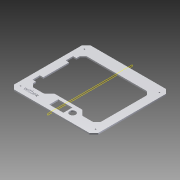
# Autodesk Inventor part: D-047
Saved by Autodesk Inventor 2015 (Build 190159000, 159)
## iProperties
Company: MARCHA TECHNOLOGY
Created: 2013-10-01
Part Number: D-047
Document SubType Name: Modeling
Designer: O.Martin
Density: 1.06 g/cm^3
Material: ABS Plastic
Mass: 736.814 g
Surface Area: 2028.63 cm^2
Volume: 695.108 cm^3
Project: WITBOXprinter_K01
Description: FRONTAL
Stock Number: 28655
Appearance: Cool White
Author: O.Martin
Autodesk Inventor part; units mm, degrees
ref_plane "XZ Plane" through (0, 0, 0) normal (0, 1, 0) x (-1, 0, 0)
ref_plane "XY Plane" through (0, 0, 0) normal (0, 0, 1) x (1, 0, 0)
sketch "Boceto1" plane through (0, 0, 0) normal (0, 0, 1) x (1, 0, 0)
  line L0 (-240, 218.25) -> (240, 218.25)
  line L1 (240, 218.25) -> (240, -218.25)
  line L2 (240, -218.25) -> (-240, -218.25)
  line L3 (-240, -218.25) -> (-240, 218.25)
  line L4 (-172.5, 153.25) -> (172.5, 153.25)
  line L5 (172.5, -153.25) -> (-172.5, -153.25)
  line L6 (-192.5, -133.25) -> (-192.5, 133.25)
  line L7 (172.5, 153.25) -> (192.5, 133.25)
  line L8 (-192.5, -133.25) -> (-172.5, -153.25)
  line L9 (-192.5, 133.25) -> (-172.5, 153.25)
  line L10 (-240, 193.25) -> (-215, 218.25)
  line L11 (240, 193.25) -> (215, 218.25)
  line L12 (-240, -193.25) -> (-215, -218.25)
  line L13 (240, -193.25) -> (215, -218.25)
  line L14 (192.5, -133.25) -> (192.5, 133.25)
  line L15 (-110, -153.25) -> (-80, -123.25)
  line L16 (-80, -123.25) -> (80, -123.25)
  line L17 (80, -123.25) -> (110, -153.25)
  line L18 (172.5, -153.25) -> (192.5, -133.25)
  point P0 (0, 0)
  point P1 (0, 218.25)
  point P2 (240, 0)
  point P3 (0, 153.25)
  point P4 (0, -123.25)
  point P5 (0, -153.25)
  point P6 (0, -218.25)
  dimension "d0" = 480
  dimension "d1" = 436.5
  dimension "d2" = 385
  dimension "d4" = 65
  dimension "d8" = 20
  dimension "d9" = 25
  dimension "d52" = 65
  dimension "d55" = 306.5
  dimension "d81" = 45
  dimension "d82" = 95
  dimension "d83" = 160
  dimension "d86" = 45
  constraints: 38 end point, 10 point on line, 7 parallel, 6 midpoint, 6 perpendicular, 5 equal length, 4 vertical alignment, 3 horizontal, 1 horizontal alignment, 1 vertical
  measures "d0" distance of L0.start L0.end
  measures "d1" distance of L0.end L1.end
  measures "d2" distance of L6.end L7.end
  measures "d4" distance between parallel lines of L2 L5
  measures "d8" horizontal distance of L6.end L4.start
  measures "d9" horizontal distance of L10.start L10.end
  measures "d52" distance between parallel lines of L0 L4
  measures "d55" distance between parallel lines of L4 L5
  measures "d81" angle of L2 L8
  measures "d82" distance between parallel lines of L2 L16
  measures "d83" distance of L15.end L16.end
  measures "d86" angle of L5 L15
extrude "Extrusión1" add sketch "Boceto1" along normal blind 8 contours L0 L11 L1 L13 L2 L12 L3 L10 | L15 L16 L17 L5
fillet "Empalme1" radius 10 12 edges at (192.5, 133.25, 4) (172.5, 153.25, 4) (-172.5, 153.25, 4) (-192.5, 133.25, 4) (-192.5, -133.25, 4) (-172.5, -153.25, 4) (-110, -153.25, 4) (110, -153.25, 4) (172.5, -153.25, 4) (192.5, -133.25, 4) (-80, -123.25, 4) (80, -123.25, 4)
sketch "Boceto3" plane through (0, 0, 8) normal (0, 0, 1) x (1, 0, 0)
  line L0 (-40.5, -141.25) -> (40.5, -141.25)
  line L1 (40.5, -141.25) -> (40.5, -192.25)
  line L2 (40.5, -192.25) -> (-40.5, -192.25)
  line L3 (-40.5, -192.25) -> (-40.5, -141.25)
  line L4 (215, -218.25) -> (-215, -218.25) projected
  line L5 (-40.5, -166.75) -> (40.5, -166.75) construction
  line L6 (0, -141.25) -> (0, -192.25) construction
  point P0 (0, -218.25)
  point P1 (0, -218.25)
  dimension "d32" = 81
  dimension "d33" = 51
  dimension "d102" = 51.5
  constraints: 12 end point, 5 midpoint, 2 parallel, 2 perpendicular, 2 vertical alignment, 1 horizontal
  measures "d32" distance of L1.end L2.end
  measures "d33" distance of L0.end L1.end
  measures "d102" distance between parallel lines of L4 L5
extrude "Extrusión3" cut sketch "Boceto3" against normal through all
sketch "Boceto8" plane through (0, 0, 8) normal (0, 0, 1) x (1, 0, 0)
  line L0 (40.5, -141.25) -> (40.5, -192.25) projected
  circle A0 centre (67.5, -166.75) radius 17.5
  line L1 (-40.5, -192.25) -> (-40.5, -141.25) projected
  line L2 (40.5, -166.75) -> (-40.5, -166.75) construction
  line L3 (-40.5, -141.25) -> (40.5, -141.25) projected
  line L4 (40.5, -192.25) -> (-40.5, -192.25) projected
  line L5 (0, -141.25) -> (0, -192.25) construction
  point P0 (190, -135.75)
  point P1 (171.2, -154.55)
  point P2 (190, -141.4069)
  dimension "d45" = 35
  dimension "d103" = 0
  dimension "d104" = 67.5
  constraints: 4 end point, 3 midpoint, 1 centre point, 2 other
  measures "d45" diameter of A0
  measures "d103" distance from line of A0.centre L2
  measures "d104" distance from line of A0.centre L5
extrude "Extrusión6" cut sketch "Boceto8" against normal through all contours A0
fillet "Empalme2" radius 1 4 edges at (-40.5, -192.25, 4) (40.5, -192.25, 4) (40.5, -141.25, 4) (-40.5, -141.25, 4)
sketch "Boceto10" plane through (0, 0, 0) normal (0, 0, -1) x (-1, 0, 0)
  line L0 (192.5, 129.1079) -> (192.5, -129.1079) projected
  line L1 (215, -218.25) -> (-215, -218.25) projected
  line L2 (192.5, 114.75) -> (211.5, 114.75)
  line L3 (211.5, 114.75) -> (211.5, 72.75)
  line L4 (211.5, 72.75) -> (192.5, 72.75)
  line L5 (192.5, 72.75) -> (192.5, 114.75)
  line L6 (192.5, -74.75) -> (211.5, -74.75)
  line L7 (211.5, -74.75) -> (211.5, -116.75)
  line L8 (211.5, -116.75) -> (192.5, -116.75)
  line L9 (192.5, -116.75) -> (192.5, -74.75)
  line L10 (211.5, -95.75) -> (192.5, -95.75) construction
  line L11 (211.5, 93.75) -> (192.5, 93.75) construction
  dimension "d60" = 42
  dimension "d61" = 122.5
  dimension "d62" = 19
  dimension "d63" = 189.5
  constraints: 20 end point, 4 midpoint, 4 parallel, 2 equal length, 2 horizontal, 2 perpendicular, 2 point on line
  measures "d60" distance of L6.end L7.end
  measures "d61" distance between parallel lines of L1 L10
  measures "d62" distance of L6.start L6.end
  measures "d63" distance between parallel lines of L10 L11
extrude "Extrusión7" cut sketch "Boceto10" against normal through all
sketch "Boceto11" plane through (0, 0, 8) normal (0, 0, 1) x (1, 0, 0)
  line L0 (-214, 182.25) -> (214, 182.25) construction
  line L1 (214, 182.25) -> (214, -182.25) construction
  line L2 (214, -182.25) -> (-214, -182.25) construction
  line L3 (-214, -182.25) -> (-214, 182.25) construction
  line L4 (-211.5, 114.75) -> (-192.5, 114.75) projected
  line L5 (-192.5, 114.75) -> (-192.5, 129.1079) projected
  arc A0 (-189.5711, 136.1789) -> (-192.5, 129.1079) centre (-182.5, 129.1079) ccw projected
  line L6 (-189.5711, 136.1789) -> (-175.4289, 150.3211) projected
  arc A1 (-168.3579, 153.25) -> (-175.4289, 150.3211) centre (-168.3579, 143.25) ccw projected
  line L7 (-168.3579, 153.25) -> (168.3579, 153.25) projected
  arc A2 (175.4289, 150.3211) -> (168.3579, 153.25) centre (168.3579, 143.25) ccw projected
  line L8 (175.4289, 150.3211) -> (189.5711, 136.1789) projected
  arc A3 (192.5, 129.1079) -> (189.5711, 136.1789) centre (182.5, 129.1079) ccw projected
  line L9 (192.5, 129.1079) -> (192.5, -129.1079) projected
  arc A4 (189.5711, -136.1789) -> (192.5, -129.1079) centre (182.5, -129.1079) ccw projected
  line L10 (189.5711, -136.1789) -> (175.4289, -150.3211) projected
  arc A5 (168.3579, -153.25) -> (175.4289, -150.3211) centre (168.3579, -143.25) ccw projected
  line L11 (168.3579, -153.25) -> (114.1421, -153.25) projected
  arc A6 (107.0711, -150.3211) -> (114.1421, -153.25) centre (114.1421, -143.25) ccw projected
  line L12 (107.0711, -150.3211) -> (82.9289, -126.1789) projected
  arc A7 (82.9289, -126.1789) -> (75.8579, -123.25) centre (75.8579, -133.25) ccw projected
  line L13 (75.8579, -123.25) -> (-75.8579, -123.25) projected
  arc A8 (-75.8579, -123.25) -> (-82.9289, -126.1789) centre (-75.8579, -133.25) ccw projected
  line L14 (-82.9289, -126.1789) -> (-107.0711, -150.3211) projected
  arc A9 (-114.1421, -153.25) -> (-107.0711, -150.3211) centre (-114.1421, -143.25) ccw projected
  line L15 (-114.1421, -153.25) -> (-168.3579, -153.25) projected
  arc A10 (-175.4289, -150.3211) -> (-168.3579, -153.25) centre (-168.3579, -143.25) ccw projected
  line L16 (-175.4289, -150.3211) -> (-189.5711, -136.1789) projected
  arc A11 (-192.5, -129.1079) -> (-189.5711, -136.1789) centre (-182.5, -129.1079) ccw projected
  line L17 (-192.5, -129.1079) -> (-192.5, -116.75) projected
  line L18 (-192.5, -116.75) -> (-211.5, -116.75) projected
  line L19 (-211.5, -116.75) -> (-211.5, -74.75) projected
  line L20 (-211.5, -74.75) -> (-192.5, -74.75) projected
  line L21 (-192.5, -74.75) -> (-192.5, 72.75) projected
  line L22 (-192.5, 72.75) -> (-211.5, 72.75) projected
  line L23 (-211.5, 72.75) -> (-211.5, 114.75) projected
  line L24 (-240, 193.25) -> (-215, 218.25) projected
  line L25 (-240, -193.25) -> (-240, 193.25) projected
  line L26 (-215, -218.25) -> (-240, -193.25) projected
  line L27 (215, -218.25) -> (-215, -218.25) projected
  line L28 (240, -193.25) -> (215, -218.25) projected
  line L29 (240, 193.25) -> (240, -193.25) projected
  line L30 (215, 218.25) -> (240, 193.25) projected
  line L31 (-215, 218.25) -> (215, 218.25) projected
  circle A12 centre (67.5, -166.75) radius 17.5 projected
  line L32 (-215, 218.25) -> (215, 218.25) projected
  point P0 (214, 0)
  point P1 (0, 182.25)
  point P2 (-214, 0)
  point P3 (214, 0)
  point P4 (0, 182.25)
  point P5 (0, -182.25)
  point P6 (0, 218.25)
  point P7 (240, 0)
  dimension "d96" = 428
  dimension "d97" = 364.5
  constraints: 8 end point, 6 coincident, 6 midpoint, 2 parallel, 1 horizontal, 1 horizontal alignment, 1 perpendicular, 1 vertical alignment
  measures "d96" distance of L0.start L0.end
  measures "d97" distance of L0.end L1.end
hole "Agujero1" at (-214, 182.25, 8) at (214, 182.25, 8) at (214, -182.25, 8) at (-214, -182.25, 8) direction (0, 0, -1) diameter 7 end through all
sketch "Boceto14" plane through (0, 0, 0) normal (0, 0, -1) x (-1, 0, 0)
  circle A0 centre (-67.5, -166.75) radius 17.5 projected
  circle A1 centre (-67.5, -148.05) radius 7.5
  dimension "d87" = 18.7
  dimension "d88" = 15
  constraints: 1 centre point, 1 vertical alignment
  measures "d87" distance of A1.centre A0.centre
  measures "d88" diameter of A1
extrude "AGUJERO BEEPER" [suppressed]
sketch "Boceto15" plane through (0, 0, 0) normal (0, 0, -1) x (-1, 0, 0)
  line L0 (215, 218.25) -> (240, 193.25) projected
  line L1 (-215, 218.25) -> (215, 218.25) projected
  line L2 (-240, 193.25) -> (-215, 218.25) projected
  line L3 (-39.5, -141.25) -> (39.5, -141.25) projected
  line L4 (-223, 210.25) -> (223, 210.25)
  dimension "d91" = 8
  constraints: 2 end point, 2 point on line, 1 parallel
  measures "d91" distance between parallel lines of L1 L4
extrude "RANURA ACOPLAMIENTO" [suppressed]
fillet "Empalme3" radius 2 4 edges at (-211.5, 114.75, 4) (-211.5, 72.75, 4) (-211.5, -74.75, 4) (-211.5, -116.75, 4)
chamfer "Chaflán5" [suppressed]
sketch "Boceto16" plane through (0, 0, 8) normal (0, 0, 1) x (1, 0, 0)
  line L0 (-240, -193.25) -> (-240, 193.25) projected
  arc A0 (-40.5, -191.25) -> (-39.5, -192.25) centre (-39.5, -191.25) ccw projected
  line L1 (-150.1777, -190.6412) -> (-150.3254, -190.6251)
  line L2 (-150.3254, -190.6251) -> (-150.4698, -190.6062)
  line L3 (-150.4698, -190.6062) -> (-150.611, -190.5846)
  line L4 (-150.611, -190.5846) -> (-150.7489, -190.56)
  line L5 (-150.7489, -190.56) -> (-150.8836, -190.5327)
  line L6 (-150.8836, -190.5327) -> (-151.015, -190.5026)
  line L7 (-151.015, -190.5026) -> (-151.1431, -190.4697)
  line L8 (-151.1431, -190.4697) -> (-151.268, -190.434)
  line L9 (-151.268, -190.434) -> (-151.3896, -190.3954)
  line L10 (-151.3896, -190.3954) -> (-151.5085, -190.3542)
  line L11 (-151.5085, -190.3542) -> (-151.6269, -190.3109)
  line L12 (-151.6269, -190.3109) -> (-151.7451, -190.2655)
  line L13 (-151.7451, -190.2655) -> (-151.8631, -190.2181)
  line L14 (-151.8631, -190.2181) -> (-151.9808, -190.1686)
  line L15 (-151.9808, -190.1686) -> (-152.0984, -190.1171)
  line L16 (-152.0984, -190.1171) -> (-152.2157, -190.0635)
  line L17 (-152.2157, -190.0635) -> (-152.3327, -190.0079)
  line L18 (-152.3327, -190.0079) -> (-152.4496, -189.9502)
  line L19 (-152.4496, -189.9502) -> (-152.5662, -189.8905)
  line L20 (-152.5662, -189.8905) -> (-152.6826, -189.8288)
  line L21 (-152.6826, -189.8288) -> (-152.7988, -189.7649)
  line L22 (-152.7988, -189.7649) -> (-152.9147, -189.6991)
  line L23 (-152.9147, -189.6991) -> (-153.0304, -189.6312)
  line L24 (-153.0304, -189.6312) -> (-153.1459, -189.5612)
  line L25 (-153.1459, -189.5612) -> (-153.3079, -190.2581)
  line L26 (-153.3079, -190.2581) -> (-155.6742, -190.2581)
  line L27 (-155.6742, -190.2581) -> (-155.6742, -169.3667)
  line L28 (-155.6742, -169.3667) -> (-153.1459, -169.3667)
  line L29 (-153.1459, -169.3667) -> (-153.1459, -176.8221)
  line L30 (-153.1459, -176.8221) -> (-153.0349, -176.7239)
  line L31 (-153.0349, -176.7239) -> (-152.9229, -176.6276)
  line L32 (-152.9229, -176.6276) -> (-152.8099, -176.5332)
  line L33 (-152.8099, -176.5332) -> (-152.6959, -176.4408)
  line L34 (-152.6959, -176.4408) -> (-152.5808, -176.3504)
  line L35 (-152.5808, -176.3504) -> (-152.4647, -176.2619)
  line L36 (-152.4647, -176.2619) -> (-152.3476, -176.1753)
  line L37 (-152.3476, -176.1753) -> (-152.2294, -176.0907)
  line L38 (-152.2294, -176.0907) -> (-152.1103, -176.008)
  line L39 (-152.1103, -176.008) -> (-151.9901, -175.9273)
  line L40 (-151.9901, -175.9273) -> (-151.8688, -175.8485)
  line L41 (-151.8688, -175.8485) -> (-151.7466, -175.7717)
  line L42 (-151.7466, -175.7717) -> (-151.6233, -175.6968)
  line L43 (-151.6233, -175.6968) -> (-151.499, -175.6238)
  line L44 (-151.499, -175.6238) -> (-151.3737, -175.5528)
  line L45 (-151.3737, -175.5528) -> (-151.2473, -175.4838)
  line L46 (-151.2473, -175.4838) -> (-151.1199, -175.4167)
  line L47 (-151.1199, -175.4167) -> (-150.9913, -175.352)
  line L48 (-150.9913, -175.352) -> (-150.8607, -175.2909)
  line L49 (-150.8607, -175.2909) -> (-150.7281, -175.2337)
  line L50 (-150.7281, -175.2337) -> (-150.5935, -175.1802)
  line L51 (-150.5935, -175.1802) -> (-150.4569, -175.1305)
  line L52 (-150.4569, -175.1305) -> (-150.3183, -175.0846)
  line L53 (-150.3183, -175.0846) -> (-150.1777, -175.0425)
  line L54 (-150.1777, -177.3465) -> (-150.3079, -177.3786)
  line L55 (-150.3079, -177.3786) -> (-150.4383, -177.4145)
  line L56 (-150.4383, -177.4145) -> (-150.569, -177.4542)
  line L57 (-150.569, -177.4542) -> (-150.7, -177.4978)
  line L58 (-150.7, -177.4978) -> (-150.8312, -177.5452)
  line L59 (-150.8312, -177.5452) -> (-150.9627, -177.5964)
  line L60 (-150.9627, -177.5964) -> (-151.0944, -177.6514)
  line L61 (-151.0944, -177.6514) -> (-151.2264, -177.7103)
  line L62 (-151.2264, -177.7103) -> (-151.3578, -177.7722)
  line L63 (-151.3578, -177.7722) -> (-151.4877, -177.8361)
  line L64 (-151.4877, -177.8361) -> (-151.6161, -177.9021)
  line L65 (-151.6161, -177.9021) -> (-151.743, -177.9701)
  line L66 (-151.743, -177.9701) -> (-151.8683, -178.0402)
  line L67 (-151.8683, -178.0402) -> (-151.9921, -178.1123)
  line L68 (-151.9921, -178.1123) -> (-152.1143, -178.1864)
  line L69 (-152.1143, -178.1864) -> (-152.2351, -178.2625)
  line L70 (-152.2351, -178.2625) -> (-152.3543, -178.3408)
  line L71 (-152.3543, -178.3408) -> (-152.472, -178.421)
  line L72 (-152.472, -178.421) -> (-152.5881, -178.5033)
  line L73 (-152.5881, -178.5033) -> (-152.7027, -178.5876)
  line L74 (-152.7027, -178.5876) -> (-152.8158, -178.674)
  line L75 (-152.8158, -178.674) -> (-152.9273, -178.7624)
  line L76 (-152.9273, -178.7624) -> (-153.0374, -178.8528)
  line L77 (-153.0374, -178.8528) -> (-153.1459, -178.9453)
  line L78 (-153.1459, -178.9453) -> (-153.1459, -187.5515)
  line L79 (-153.1459, -187.5515) -> (-153.0034, -187.6206)
  line L80 (-153.0034, -187.6206) -> (-152.8633, -187.6865)
  line L81 (-152.8633, -187.6865) -> (-152.7258, -187.7494)
  line L82 (-152.7258, -187.7494) -> (-152.5907, -187.8092)
  line L83 (-152.5907, -187.8092) -> (-152.4581, -187.8658)
  line L84 (-152.4581, -187.8658) -> (-152.3279, -187.9193)
  line L85 (-152.3279, -187.9193) -> (-152.2003, -187.9698)
  line L86 (-152.2003, -187.9698) -> (-152.0751, -188.0171)
  line L87 (-152.0751, -188.0171) -> (-151.9523, -188.0612)
  line L88 (-151.9523, -188.0612) -> (-151.8321, -188.1023)
  line L89 (-151.8321, -188.1023) -> (-151.7143, -188.1403)
  line L90 (-151.7143, -188.1403) -> (-151.599, -188.1752)
  line L91 (-151.599, -188.1752) -> (-151.4861, -188.2069)
  line L92 (-151.4861, -188.2069) -> (-151.3748, -188.2357)
  line L93 (-151.3748, -188.2357) -> (-151.2621, -188.2624)
  line L94 (-151.2621, -188.2624) -> (-151.1478, -188.2868)
  line L95 (-151.1478, -188.2868) -> (-151.032, -188.309)
  line L96 (-151.032, -188.309) -> (-150.9146, -188.329)
  line L97 (-150.9146, -188.329) -> (-150.7957, -188.3468)
  line L98 (-150.7957, -188.3468) -> (-150.6752, -188.3624)
  line L99 (-150.6752, -188.3624) -> (-150.5532, -188.3759)
  line L100 (-150.5532, -188.3759) -> (-150.4296, -188.3871)
  line L101 (-150.4296, -188.3871) -> (-150.3044, -188.3961)
  line L102 (-150.3044, -188.3961) -> (-150.1777, -188.403)
  line L103 (-135.7538, -177.0885) -> (-136.0028, -177.1477)
  line L104 (-136.0028, -177.1477) -> (-136.2422, -177.2219)
  line L105 (-136.2422, -177.2219) -> (-136.4722, -177.3112)
  line L106 (-136.4722, -177.3112) -> (-136.6927, -177.4156)
  line L107 (-136.6927, -177.4156) -> (-136.9037, -177.5351)
  line L108 (-136.9037, -177.5351) -> (-137.1052, -177.6697)
  line L109 (-137.1052, -177.6697) -> (-137.2972, -177.8194)
  line L110 (-137.2972, -177.8194) -> (-137.4798, -177.9841)
  line L111 (-137.4798, -177.9841) -> (-137.6528, -178.164)
  line L112 (-137.6528, -178.164) -> (-137.8164, -178.3589)
  line L113 (-137.8164, -178.3589) -> (-137.97, -178.5692)
  line L114 (-137.97, -178.5692) -> (-138.1123, -178.7954)
  line L115 (-138.1123, -178.7954) -> (-138.2432, -179.0375)
  line L116 (-138.2432, -179.0375) -> (-138.3627, -179.2956)
  line L117 (-138.3627, -179.2956) -> (-138.4709, -179.5697)
  line L118 (-138.4709, -179.5697) -> (-138.5676, -179.8597)
  line L119 (-138.5676, -179.8597) -> (-138.653, -180.1656)
  line L120 (-138.653, -180.1656) -> (-138.727, -180.4875)
  line L121 (-138.727, -180.4875) -> (-138.7896, -180.8254)
  line L122 (-138.7896, -180.8254) -> (-138.8409, -181.1792)
  line L123 (-138.8409, -181.1792) -> (-138.8807, -181.549)
  line L124 (-138.8807, -181.549) -> (-138.9092, -181.9347)
  line L125 (-138.9092, -181.9347) -> (-138.9262, -182.3364)
  line L126 (-138.9262, -182.3364) -> (-138.9319, -182.7541)
  line L127 (-138.9319, -182.7541) -> (-138.9262, -183.1605)
  line L128 (-138.9262, -183.1605) -> (-138.9092, -183.5523)
  line L129 (-138.9092, -183.5523) -> (-138.8807, -183.9295)
  line L130 (-138.8807, -183.9295) -> (-138.8409, -184.2919)
  line L131 (-138.8409, -184.2919) -> (-138.7896, -184.6398)
  line L132 (-138.7896, -184.6398) -> (-138.727, -184.9729)
  line L133 (-138.727, -184.9729) -> (-138.653, -185.2914)
  line L134 (-138.653, -185.2914) -> (-138.5676, -185.5952)
  line L135 (-138.5676, -185.5952) -> (-138.4709, -185.8844)
  line L136 (-138.4709, -185.8844) -> (-138.3627, -186.1589)
  line L137 (-138.3627, -186.1589) -> (-138.2432, -186.4188)
  line L138 (-138.2432, -186.4188) -> (-138.1123, -186.664)
  line L139 (-138.1123, -186.664) -> (-137.97, -186.8945)
  line L140 (-137.97, -186.8945) -> (-137.8164, -187.1103)
  line L141 (-137.8164, -187.1103) -> (-137.6528, -187.3109)
  line L142 (-137.6528, -187.3109) -> (-137.4798, -187.4959)
  line L143 (-137.4798, -187.4959) -> (-137.2972, -187.6653)
  line L144 (-137.2972, -187.6653) -> (-137.1052, -187.8193)
  line L145 (-137.1052, -187.8193) -> (-136.9037, -187.9577)
  line L146 (-136.9037, -187.9577) -> (-136.6927, -188.0806)
  line L147 (-136.6927, -188.0806) -> (-136.4722, -188.188)
  line L148 (-136.4722, -188.188) -> (-136.2422, -188.2799)
  line L149 (-136.2422, -188.2799) -> (-136.0028, -188.3562)
  line L150 (-136.0028, -188.3562) -> (-135.7538, -188.417)
  line L151 (-135.7538, -190.63) -> (-136.1962, -190.5674)
  line L152 (-136.1962, -190.5674) -> (-136.6226, -190.4794)
  line L153 (-136.6226, -190.4794) -> (-137.0332, -190.3663)
  line L154 (-137.0332, -190.3663) -> (-137.428, -190.2279)
  line L155 (-137.428, -190.2279) -> (-137.8069, -190.0642)
  line L156 (-137.8069, -190.0642) -> (-138.17, -189.8752)
  line L157 (-138.17, -189.8752) -> (-138.5172, -189.661)
  line L158 (-138.5172, -189.661) -> (-138.8486, -189.4215)
  line L159 (-138.8486, -189.4215) -> (-139.1641, -189.1568)
  line L160 (-139.1641, -189.1568) -> (-139.4638, -188.8668)
  line L161 (-139.4638, -188.8668) -> (-139.7476, -188.5515)
  line L162 (-139.7476, -188.5515) -> (-140.013, -188.2145)
  line L163 (-140.013, -188.2145) -> (-140.2571, -187.8593)
  line L164 (-140.2571, -187.8593) -> (-140.48, -187.486)
  line L165 (-140.48, -187.486) -> (-140.6816, -187.0945)
  line L166 (-140.6816, -187.0945) -> (-140.8621, -186.6848)
  line L167 (-140.8621, -186.6848) -> (-141.0213, -186.257)
  line L168 (-141.0213, -186.257) -> (-141.1592, -185.811)
  line L169 (-141.1592, -185.811) -> (-141.276, -185.3469)
  line L170 (-141.276, -185.3469) -> (-141.3715, -184.8647)
  line L171 (-141.3715, -184.8647) -> (-141.4458, -184.3642)
  line L172 (-141.4458, -184.3642) -> (-141.4989, -183.8457)
  line L173 (-141.4989, -183.8457) -> (-141.5307, -183.3089)
  line L174 (-141.5307, -183.3089) -> (-141.5413, -182.7541)
  line L175 (-141.5413, -182.7541) -> (-141.5304, -182.1867)
  line L176 (-141.5304, -182.1867) -> (-141.4978, -181.6391)
  line L177 (-141.4978, -181.6391) -> (-141.4434, -181.1113)
  line L178 (-141.4434, -181.1113) -> (-141.3672, -180.6032)
  line L179 (-141.3672, -180.6032) -> (-141.2692, -180.1149)
  line L180 (-141.2692, -180.1149) -> (-141.1494, -179.6464)
  line L181 (-141.1494, -179.6464) -> (-141.0079, -179.1977)
  line L182 (-141.0079, -179.1977) -> (-140.8446, -178.7687)
  line L183 (-140.8446, -178.7687) -> (-140.6596, -178.3594)
  line L184 (-140.6596, -178.3594) -> (-140.4527, -177.97)
  line L185 (-140.4527, -177.97) -> (-140.2241, -177.6003)
  line L186 (-140.2241, -177.6003) -> (-139.9738, -177.2504)
  line L187 (-139.9738, -177.2504) -> (-139.7016, -176.9202)
  line L188 (-139.7016, -176.9202) -> (-139.4115, -176.6121)
  line L189 (-139.4115, -176.6121) -> (-139.1076, -176.3285)
  line L190 (-139.1076, -176.3285) -> (-138.79, -176.0694)
  line L191 (-138.79, -176.0694) -> (-138.4586, -175.8349)
  line L192 (-138.4586, -175.8349) -> (-138.1134, -175.6249)
  line L193 (-138.1134, -175.6249) -> (-137.7545, -175.4395)
  line L194 (-137.7545, -175.4395) -> (-137.3819, -175.2786)
  line L195 (-137.3819, -175.2786) -> (-136.9955, -175.1423)
  line L196 (-136.9955, -175.1423) -> (-136.5954, -175.0305)
  line L197 (-136.5954, -175.0305) -> (-136.1815, -174.9432)
  line L198 (-136.1815, -174.9432) -> (-135.7538, -174.8805)
  line L199 (-175.9335, -175.25) -> (-173.389, -175.25)
  line L200 (-173.389, -175.25) -> (-177.1977, -190.2581)
  line L201 (-177.1977, -190.2581) -> (-179.5316, -190.2581)
  line L202 (-179.5316, -190.2581) -> (-183.1945, -178.686)
  line L203 (-183.1945, -178.686) -> (-186.8412, -190.2581)
  line L204 (-186.8412, -190.2581) -> (-189.1588, -190.2581)
  line L205 (-189.1588, -190.2581) -> (-193, -175.25)
  line L206 (-193, -175.25) -> (-190.3744, -175.25)
  line L207 (-190.3744, -175.25) -> (-187.7164, -186.8707)
  line L208 (-187.7164, -186.8707) -> (-184.1669, -175.25)
  line L209 (-184.1669, -175.25) -> (-182.0762, -175.25)
  line L210 (-182.0762, -175.25) -> (-178.4295, -186.8707)
  line L211 (-178.4295, -186.8707) -> (-175.9335, -175.25)
  line L212 (-168.5916, -175.25) -> (-168.5916, -190.2581)
  line L213 (-168.5916, -190.2581) -> (-171.1199, -190.2581)
  line L214 (-171.1199, -190.2581) -> (-171.1199, -175.25)
  line L215 (-171.1199, -175.25) -> (-168.5916, -175.25)
  line L216 (-168.4133, -170.1284) -> (-168.4133, -172.7541)
  line L217 (-168.4133, -172.7541) -> (-171.282, -172.7541)
  line L218 (-171.282, -172.7541) -> (-171.282, -170.1284)
  line L219 (-171.282, -170.1284) -> (-168.4133, -170.1284)
  line L220 (-157.5381, -190.1284) -> (-157.6571, -190.1603)
  line L221 (-157.6571, -190.1603) -> (-157.7762, -190.191)
  line L222 (-157.7762, -190.191) -> (-157.8957, -190.2206)
  line L223 (-157.8957, -190.2206) -> (-158.0153, -190.2491)
  line L224 (-158.0153, -190.2491) -> (-158.1352, -190.2764)
  line L225 (-158.1352, -190.2764) -> (-158.2553, -190.3027)
  line L226 (-158.2553, -190.3027) -> (-158.3756, -190.3278)
  line L227 (-158.3756, -190.3278) -> (-158.4961, -190.3517)
  line L228 (-158.4961, -190.3517) -> (-158.6169, -190.3746)
  line L229 (-158.6169, -190.3746) -> (-158.7379, -190.3963)
  line L230 (-158.7379, -190.3963) -> (-158.8591, -190.4169)
  line L231 (-158.8591, -190.4169) -> (-158.9806, -190.4364)
  line L232 (-158.9806, -190.4364) -> (-159.1014, -190.4545)
  line L233 (-159.1014, -190.4545) -> (-159.221, -190.4711)
  line L234 (-159.221, -190.4711) -> (-159.3391, -190.486)
  line L235 (-159.3391, -190.486) -> (-159.456, -190.4994)
  line L236 (-159.456, -190.4994) -> (-159.5714, -190.5112)
  line L237 (-159.5714, -190.5112) -> (-159.6856, -190.5215)
  line L238 (-159.6856, -190.5215) -> (-159.7984, -190.5301)
  line L239 (-159.7984, -190.5301) -> (-159.9098, -190.5372)
  line L240 (-159.9098, -190.5372) -> (-160.0199, -190.5427)
  line L241 (-160.0199, -190.5427) -> (-160.1286, -190.5467)
  line L242 (-160.1286, -190.5467) -> (-160.236, -190.549)
  line L243 (-160.236, -190.549) -> (-160.342, -190.5498)
  line L244 (-160.342, -190.5498) -> (-160.6788, -190.5417)
  line L245 (-160.6788, -190.5417) -> (-161.0031, -190.5172)
  line L246 (-161.0031, -190.5172) -> (-161.3149, -190.4764)
  line L247 (-161.3149, -190.4764) -> (-161.6143, -190.4193)
  line L248 (-161.6143, -190.4193) -> (-161.9011, -190.3458)
  line L249 (-161.9011, -190.3458) -> (-162.1754, -190.2561)
  line L250 (-162.1754, -190.2561) -> (-162.4373, -190.15)
  line L251 (-162.4373, -190.15) -> (-162.6867, -190.0276)
  line L252 (-162.6867, -190.0276) -> (-162.9235, -189.8889)
  line L253 (-162.9235, -189.8889) -> (-163.1479, -189.7338)
  line L254 (-163.1479, -189.7338) -> (-163.3598, -189.5625)
  line L255 (-163.3598, -189.5625) -> (-163.5592, -189.3748)
  line L256 (-163.5592, -189.3748) -> (-163.7442, -189.1694)
  line L257 (-163.7442, -189.1694) -> (-163.9132, -188.9451)
  line L258 (-163.9132, -188.9451) -> (-164.0661, -188.7017)
  line L259 (-164.0661, -188.7017) -> (-164.203, -188.4393)
  line L260 (-164.203, -188.4393) -> (-164.3237, -188.1578)
  line L261 (-164.3237, -188.1578) -> (-164.4283, -187.8574)
  line L262 (-164.4283, -187.8574) -> (-164.5168, -187.5379)
  line L263 (-164.5168, -187.5379) -> (-164.5892, -187.1994)
  line L264 (-164.5892, -187.1994) -> (-164.6456, -186.8419)
  line L265 (-164.6456, -186.8419) -> (-164.6858, -186.4653)
  line L266 (-164.6858, -186.4653) -> (-164.7099, -186.0698)
  line L267 (-164.7099, -186.0698) -> (-164.718, -185.6552)
  line L268 (-164.718, -185.6552) -> (-164.718, -177.3408)
  line L269 (-164.718, -177.3408) -> (-166.4198, -177.3408)
  line L270 (-166.4198, -177.3408) -> (-166.4198, -175.25)
  line L271 (-166.4198, -175.25) -> (-164.718, -175.25)
  line L272 (-164.718, -175.25) -> (-164.718, -170.9388)
  line L273 (-164.718, -170.9388) -> (-162.1896, -170.9388)
  line L274 (-162.1896, -170.9388) -> (-162.1896, -175.25)
  line L275 (-162.1896, -175.25) -> (-157.5381, -175.25)
  line L276 (-157.5381, -175.25) -> (-157.5381, -177.3408)
  line L277 (-157.5381, -177.3408) -> (-162.1896, -177.3408)
  line L278 (-162.1896, -177.3408) -> (-162.1896, -184.4883)
  line L279 (-162.1896, -184.4883) -> (-162.1893, -184.6738)
  line L280 (-162.1893, -184.6738) -> (-162.1885, -184.8522)
  line L281 (-162.1885, -184.8522) -> (-162.1871, -185.0236)
  line L282 (-162.1871, -185.0236) -> (-162.1851, -185.1879)
  line L283 (-162.1851, -185.1879) -> (-162.1826, -185.3451)
  line L284 (-162.1826, -185.3451) -> (-162.1795, -185.4951)
  line L285 (-162.1795, -185.4951) -> (-162.1758, -185.6381)
  line L286 (-162.1758, -185.6381) -> (-162.1716, -185.774)
  line L287 (-162.1716, -185.774) -> (-162.1668, -185.9029)
  line L288 (-162.1668, -185.9029) -> (-162.1615, -186.0246)
  line L289 (-162.1615, -186.0246) -> (-162.1556, -186.1392)
  line L290 (-162.1556, -186.1392) -> (-162.1491, -186.2468)
  line L291 (-162.1491, -186.2468) -> (-162.1407, -186.3501)
  line L292 (-162.1407, -186.3501) -> (-162.1291, -186.4523)
  line L293 (-162.1291, -186.4523) -> (-162.1142, -186.5532)
  line L294 (-162.1142, -186.5532) -> (-162.096, -186.6528)
  line L295 (-162.096, -186.6528) -> (-162.0745, -186.7513)
  line L296 (-162.0745, -186.7513) -> (-162.0498, -186.8485)
  line L297 (-162.0498, -186.8485) -> (-162.0219, -186.9444)
  line L298 (-162.0219, -186.9444) -> (-161.9906, -187.0391)
  line L299 (-161.9906, -187.0391) -> (-161.9561, -187.1326)
  line L300 (-161.9561, -187.1326) -> (-161.9184, -187.2248)
  line L301 (-161.9184, -187.2248) -> (-161.8774, -187.3158)
  line L302 (-161.8774, -187.3158) -> (-161.8331, -187.4056)
  line L303 (-161.8331, -187.4056) -> (-161.7933, -187.4823)
  line L304 (-161.7933, -187.4823) -> (-161.7495, -187.5557)
  line L305 (-161.7495, -187.5557) -> (-161.7019, -187.6259)
  line L306 (-161.7019, -187.6259) -> (-161.6503, -187.6928)
  line L307 (-161.6503, -187.6928) -> (-161.5947, -187.7565)
  line L308 (-161.5947, -187.7565) -> (-161.5353, -187.8169)
  line L309 (-161.5353, -187.8169) -> (-161.4718, -187.874)
  line L310 (-161.4718, -187.874) -> (-161.4045, -187.9278)
  line L311 (-161.4045, -187.9278) -> (-161.3332, -187.9784)
  line L312 (-161.3332, -187.9784) -> (-161.2579, -188.0258)
  line L313 (-161.2579, -188.0258) -> (-161.1787, -188.0698)
  line L314 (-161.1787, -188.0698) -> (-161.0956, -188.1106)
  line L315 (-161.0956, -188.1106) -> (-161.008, -188.1482)
  line L316 (-161.008, -188.1482) -> (-160.9153, -188.1824)
  line L317 (-160.9153, -188.1824) -> (-160.8176, -188.2134)
  line L318 (-160.8176, -188.2134) -> (-160.7147, -188.2412)
  line L319 (-160.7147, -188.2412) -> (-160.6069, -188.2657)
  line L320 (-160.6069, -188.2657) -> (-160.4939, -188.2869)
  line L321 (-160.4939, -188.2869) -> (-160.3759, -188.3048)
  line L322 (-160.3759, -188.3048) -> (-160.2528, -188.3195)
  line L323 (-160.2528, -188.3195) -> (-160.1247, -188.3309)
  line L324 (-160.1247, -188.3309) -> (-159.9915, -188.3391)
  line L325 (-159.9915, -188.3391) -> (-159.8532, -188.344)
  line L326 (-159.8532, -188.344) -> (-159.7099, -188.3456)
  line L327 (-159.7099, -188.3456) -> (-159.6075, -188.3443)
  line L328 (-159.6075, -188.3443) -> (-159.5057, -188.3404)
  line L329 (-159.5057, -188.3404) -> (-159.4045, -188.334)
  line L330 (-159.4045, -188.334) -> (-159.3038, -188.3249)
  line L331 (-159.3038, -188.3249) -> (-159.2037, -188.3133)
  line L332 (-159.2037, -188.3133) -> (-159.1041, -188.299)
  line L333 (-159.1041, -188.299) -> (-159.0051, -188.2822)
  line L334 (-159.0051, -188.2822) -> (-158.9067, -188.2628)
  line L335 (-158.9067, -188.2628) -> (-158.8089, -188.2408)
  line L336 (-158.8089, -188.2408) -> (-158.7116, -188.2162)
  line L337 (-158.7116, -188.2162) -> (-158.6148, -188.189)
  line L338 (-158.6148, -188.189) -> (-158.5186, -188.1592)
  line L339 (-158.5186, -188.1592) -> (-158.4249, -188.1287)
  line L340 (-158.4249, -188.1287) -> (-158.3356, -188.0991)
  line L341 (-158.3356, -188.0991) -> (-158.2507, -188.0706)
  line L342 (-158.2507, -188.0706) -> (-158.1702, -188.0431)
  line L343 (-158.1702, -188.0431) -> (-158.094, -188.0166)
  line L344 (-158.094, -188.0166) -> (-158.0223, -187.9911)
  line L345 (-158.0223, -187.9911) -> (-157.9549, -187.9666)
  line L346 (-157.9549, -187.9666) -> (-157.892, -187.9431)
  line L347 (-157.892, -187.9431) -> (-157.8334, -187.9207)
  line L348 (-157.8334, -187.9207) -> (-157.7792, -187.8992)
  line L349 (-157.7792, -187.8992) -> (-157.7294, -187.8788)
  line L350 (-157.7294, -187.8788) -> (-157.684, -187.8594)
  line L351 (-157.684, -187.8594) -> (-157.5381, -187.8594)
  line L352 (-157.5381, -187.8594) -> (-157.5381, -190.1284)
  line L353 (-148.1777, -188.0946) -> (-147.987, -188.0058)
  line L354 (-147.987, -188.0058) -> (-147.803, -187.906)
  line L355 (-147.803, -187.906) -> (-147.6256, -187.7953)
  line L356 (-147.6256, -187.7953) -> (-147.4548, -187.6735)
  line L357 (-147.4548, -187.6735) -> (-147.2906, -187.5408)
  line L358 (-147.2906, -187.5408) -> (-147.1331, -187.3971)
  line L359 (-147.1331, -187.3971) -> (-146.9822, -187.2424)
  line L360 (-146.9822, -187.2424) -> (-146.8379, -187.0768)
  line L361 (-146.8379, -187.0768) -> (-146.701, -186.8995)
  line L362 (-146.701, -186.8995) -> (-146.5728, -186.7095)
  line L363 (-146.5728, -186.7095) -> (-146.4535, -186.5068)
  line L364 (-146.4535, -186.5068) -> (-146.343, -186.2912)
  line L365 (-146.343, -186.2912) -> (-146.2414, -186.0628)
  line L366 (-146.2414, -186.0628) -> (-146.1486, -185.8216)
  line L367 (-146.1486, -185.8216) -> (-146.0646, -185.5676)
  line L368 (-146.0646, -185.5676) -> (-145.9895, -185.3008)
  line L369 (-145.9895, -185.3008) -> (-145.9232, -185.0212)
  line L370 (-145.9232, -185.0212) -> (-145.8657, -184.7287)
  line L371 (-145.8657, -184.7287) -> (-145.8171, -184.4235)
  line L372 (-145.8171, -184.4235) -> (-145.7774, -184.1055)
  line L373 (-145.7774, -184.1055) -> (-145.7464, -183.7747)
  line L374 (-145.7464, -183.7747) -> (-145.7243, -183.4311)
  line L375 (-145.7243, -183.4311) -> (-145.7111, -183.0747)
  line L376 (-145.7111, -183.0747) -> (-145.7066, -182.7054)
  line L377 (-145.7066, -182.7054) -> (-145.7108, -182.3295)
  line L378 (-145.7108, -182.3295) -> (-145.7232, -181.9666)
  line L379 (-145.7232, -181.9666) -> (-145.7439, -181.6169)
  line L380 (-145.7439, -181.6169) -> (-145.7728, -181.2803)
  line L381 (-145.7728, -181.2803) -> (-145.81, -180.9567)
  line L382 (-145.81, -180.9567) -> (-145.8555, -180.6463)
  line L383 (-145.8555, -180.6463) -> (-145.9093, -180.349)
  line L384 (-145.9093, -180.349) -> (-145.9713, -180.0648)
  line L385 (-145.9713, -180.0648) -> (-146.0416, -179.7937)
  line L386 (-146.0416, -179.7937) -> (-146.1202, -179.5356)
  line L387 (-146.1202, -179.5356) -> (-146.2071, -179.2907)
  line L388 (-146.2071, -179.2907) -> (-146.3022, -179.0589)
  line L389 (-146.3022, -179.0589) -> (-146.4056, -178.8402)
  line L390 (-146.4056, -178.8402) -> (-146.5172, -178.6346)
  line L391 (-146.5172, -178.6346) -> (-146.638, -178.4426)
  line L392 (-146.638, -178.4426) -> (-146.7688, -178.2646)
  line L393 (-146.7688, -178.2646) -> (-146.9096, -178.1007)
  line L394 (-146.9096, -178.1007) -> (-147.0606, -177.9509)
  line L395 (-147.0606, -177.9509) -> (-147.2216, -177.8151)
  line L396 (-147.2216, -177.8151) -> (-147.3926, -177.6935)
  line L397 (-147.3926, -177.6935) -> (-147.5738, -177.5859)
  line L398 (-147.5738, -177.5859) -> (-147.765, -177.4925)
  line L399 (-147.765, -177.4925) -> (-147.9663, -177.4131)
  line L400 (-147.9663, -177.4131) -> (-148.1777, -177.3478)
  line L401 (-148.1777, -174.8404) -> (-147.79, -174.8783)
  line L402 (-147.79, -174.8783) -> (-147.4163, -174.9424)
  line L403 (-147.4163, -174.9424) -> (-147.0565, -175.0326)
  line L404 (-147.0565, -175.0326) -> (-146.7106, -175.1489)
  line L405 (-146.7106, -175.1489) -> (-146.3788, -175.2914)
  line L406 (-146.3788, -175.2914) -> (-146.0608, -175.46)
  line L407 (-146.0608, -175.46) -> (-145.7569, -175.6547)
  line L408 (-145.7569, -175.6547) -> (-145.4669, -175.8756)
  line L409 (-145.4669, -175.8756) -> (-145.1908, -176.1227)
  line L410 (-145.1908, -176.1227) -> (-144.9287, -176.3958)
  line L411 (-144.9287, -176.3958) -> (-144.6805, -176.6951)
  line L412 (-144.6805, -176.6951) -> (-144.4469, -177.0199)
  line L413 (-144.4469, -177.0199) -> (-144.2313, -177.3658)
  line L414 (-144.2313, -177.3658) -> (-144.0345, -177.732)
  line L415 (-144.0345, -177.732) -> (-143.8564, -178.1185)
  line L416 (-143.8564, -178.1185) -> (-143.6971, -178.5253)
  line L417 (-143.6971, -178.5253) -> (-143.5565, -178.9525)
  line L418 (-143.5565, -178.9525) -> (-143.4347, -179.3999)
  line L419 (-143.4347, -179.3999) -> (-143.3316, -179.8676)
  line L420 (-143.3316, -179.8676) -> (-143.2472, -180.3557)
  line L421 (-143.2472, -180.3557) -> (-143.1816, -180.864)
  line L422 (-143.1816, -180.864) -> (-143.1347, -181.3927)
  line L423 (-143.1347, -181.3927) -> (-143.1066, -181.9417)
  line L424 (-143.1066, -181.9417) -> (-143.0972, -182.5109)
  line L425 (-143.0972, -182.5109) -> (-143.107, -183.0466)
  line L426 (-143.107, -183.0466) -> (-143.1362, -183.5667)
  line L427 (-143.1362, -183.5667) -> (-143.1848, -184.0711)
  line L428 (-143.1848, -184.0711) -> (-143.2529, -184.5598)
  line L429 (-143.2529, -184.5598) -> (-143.3404, -185.0329)
  line L430 (-143.3404, -185.0329) -> (-143.4474, -185.4904)
  line L431 (-143.4474, -185.4904) -> (-143.5739, -185.9321)
  line L432 (-143.5739, -185.9321) -> (-143.7198, -186.3583)
  line L433 (-143.7198, -186.3583) -> (-143.8852, -186.7688)
  line L434 (-143.8852, -186.7688) -> (-144.07, -187.1636)
  line L435 (-144.07, -187.1636) -> (-144.2743, -187.5428)
  line L436 (-144.2743, -187.5428) -> (-144.498, -187.9063)
  line L437 (-144.498, -187.9063) -> (-144.7412, -188.2541)
  line L438 (-144.7412, -188.2541) -> (-145.0029, -188.5854)
  line L439 (-145.0029, -188.5854) -> (-145.2758, -188.8935)
  line L440 (-145.2758, -188.8935) -> (-145.5586, -189.177)
  line L441 (-145.5586, -189.177) -> (-145.8513, -189.4361)
  line L442 (-145.8513, -189.4361) -> (-146.1539, -189.6707)
  line L443 (-146.1539, -189.6707) -> (-146.4665, -189.8807)
  line L444 (-146.4665, -189.8807) -> (-146.7889, -190.0663)
  line L445 (-146.7889, -190.0663) -> (-147.1212, -190.2274)
  line L446 (-147.1212, -190.2274) -> (-147.4635, -190.364)
  line L447 (-147.4635, -190.364) -> (-147.8156, -190.476)
  line L448 (-147.8156, -190.476) -> (-148.1777, -190.5636)
  line L449 (-119.0616, -182.6568) -> (-113.8914, -190.2581)
  line L450 (-113.8914, -190.2581) -> (-116.987, -190.2581)
  line L451 (-116.987, -190.2581) -> (-120.6337, -184.6179)
  line L452 (-120.6337, -184.6179) -> (-124.3776, -190.2581)
  line L453 (-124.3776, -190.2581) -> (-127.2464, -190.2581)
  line L454 (-127.2464, -190.2581) -> (-122.0438, -182.8189)
  line L455 (-122.0438, -182.8189) -> (-127.1977, -175.25)
  line L456 (-127.1977, -175.25) -> (-124.1021, -175.25)
  line L457 (-124.1021, -175.25) -> (-120.4716, -180.8416)
  line L458 (-120.4716, -180.8416) -> (-116.7601, -175.25)
  line L459 (-116.7601, -175.25) -> (-113.8914, -175.25)
  line L460 (-113.8914, -175.25) -> (-119.0616, -182.6568)
  line L461 (-133.7538, -174.8985) -> (-133.3336, -174.9681)
  line L462 (-133.3336, -174.9681) -> (-132.9275, -175.0614)
  line L463 (-132.9275, -175.0614) -> (-132.5353, -175.1784)
  line L464 (-132.5353, -175.1784) -> (-132.1572, -175.3193)
  line L465 (-132.1572, -175.3193) -> (-131.793, -175.4839)
  line L466 (-131.793, -175.4839) -> (-131.4429, -175.6722)
  line L467 (-131.4429, -175.6722) -> (-131.1068, -175.8844)
  line L468 (-131.1068, -175.8844) -> (-130.7848, -176.1203)
  line L469 (-130.7848, -176.1203) -> (-130.4767, -176.3799)
  line L470 (-130.4767, -176.3799) -> (-130.1827, -176.6634)
  line L471 (-130.1827, -176.6634) -> (-129.9028, -176.9705)
  line L472 (-129.9028, -176.9705) -> (-129.6417, -177.2984)
  line L473 (-129.6417, -177.2984) -> (-129.4015, -177.6458)
  line L474 (-129.4015, -177.6458) -> (-129.1822, -178.0127)
  line L475 (-129.1822, -178.0127) -> (-128.9837, -178.3991)
  line L476 (-128.9837, -178.3991) -> (-128.8062, -178.805)
  line L477 (-128.8062, -178.805) -> (-128.6495, -179.2304)
  line L478 (-128.6495, -179.2304) -> (-128.5137, -179.6753)
  line L479 (-128.5137, -179.6753) -> (-128.3989, -180.1397)
  line L480 (-128.3989, -180.1397) -> (-128.3049, -180.6236)
  line L481 (-128.3049, -180.6236) -> (-128.2318, -181.1269)
  line L482 (-128.2318, -181.1269) -> (-128.1795, -181.6498)
  line L483 (-128.1795, -181.6498) -> (-128.1482, -182.1922)
  line L484 (-128.1482, -182.1922) -> (-128.1378, -182.7541)
  line L485 (-128.1378, -182.7541) -> (-128.1482, -183.3182)
  line L486 (-128.1482, -183.3182) -> (-128.1795, -183.8626)
  line L487 (-128.1795, -183.8626) -> (-128.2318, -184.3873)
  line L488 (-128.2318, -184.3873) -> (-128.3049, -184.8921)
  line L489 (-128.3049, -184.8921) -> (-128.3989, -185.3772)
  line L490 (-128.3989, -185.3772) -> (-128.5137, -185.8425)
  line L491 (-128.5137, -185.8425) -> (-128.6495, -186.288)
  line L492 (-128.6495, -186.288) -> (-128.8062, -186.7138)
  line L493 (-128.8062, -186.7138) -> (-128.9837, -187.1198)
  line L494 (-128.9837, -187.1198) -> (-129.1822, -187.506)
  line L495 (-129.1822, -187.506) -> (-129.4015, -187.8724)
  line L496 (-129.4015, -187.8724) -> (-129.6417, -188.2191)
  line L497 (-129.6417, -188.2191) -> (-129.9028, -188.546)
  line L498 (-129.9028, -188.546) -> (-130.1827, -188.8519)
  line L499 (-130.1827, -188.8519) -> (-130.4767, -189.1342)
  line L500 (-130.4767, -189.1342) -> (-130.7848, -189.3929)
  line L501 (-130.7848, -189.3929) -> (-131.1068, -189.6279)
  line L502 (-131.1068, -189.6279) -> (-131.4429, -189.8392)
  line L503 (-131.4429, -189.8392) -> (-131.793, -190.0268)
  line L504 (-131.793, -190.0268) -> (-132.1572, -190.1907)
  line L505 (-132.1572, -190.1907) -> (-132.5353, -190.331)
  line L506 (-132.5353, -190.331) -> (-132.9275, -190.4476)
  line L507 (-132.9275, -190.4476) -> (-133.3336, -190.5406)
  line L508 (-133.3336, -190.5406) -> (-133.7538, -190.6098)
  line L509 (-133.7538, -188.3813) -> (-133.5191, -188.3136)
  line L510 (-133.5191, -188.3136) -> (-133.2932, -188.2315)
  line L511 (-133.2932, -188.2315) -> (-133.076, -188.135)
  line L512 (-133.076, -188.135) -> (-132.8677, -188.024)
  line L513 (-132.8677, -188.024) -> (-132.6682, -187.8985)
  line L514 (-132.6682, -187.8985) -> (-132.4775, -187.7587)
  line L515 (-132.4775, -187.7587) -> (-132.2957, -187.6043)
  line L516 (-132.2957, -187.6043) -> (-132.1226, -187.4355)
  line L517 (-132.1226, -187.4355) -> (-131.9584, -187.2523)
  line L518 (-131.9584, -187.2523) -> (-131.803, -187.0546)
  line L519 (-131.803, -187.0546) -> (-131.6575, -186.8424)
  line L520 (-131.6575, -186.8424) -> (-131.5229, -186.6156)
  line L521 (-131.5229, -186.6156) -> (-131.399, -186.3741)
  line L522 (-131.399, -186.3741) -> (-131.2859, -186.1181)
  line L523 (-131.2859, -186.1181) -> (-131.1835, -185.8474)
  line L524 (-131.1835, -185.8474) -> (-131.0919, -185.5622)
  line L525 (-131.0919, -185.5622) -> (-131.0111, -185.2623)
  line L526 (-131.0111, -185.2623) -> (-130.9411, -184.9478)
  line L527 (-130.9411, -184.9478) -> (-130.8818, -184.6187)
  line L528 (-130.8818, -184.6187) -> (-130.8334, -184.275)
  line L529 (-130.8334, -184.275) -> (-130.7956, -183.9167)
  line L530 (-130.7956, -183.9167) -> (-130.7687, -183.5437)
  line L531 (-130.7687, -183.5437) -> (-130.7526, -183.1562)
  line L532 (-130.7526, -183.1562) -> (-130.7472, -182.7541)
  line L533 (-130.7472, -182.7541) -> (-130.7525, -182.347)
  line L534 (-130.7525, -182.347) -> (-130.7686, -181.9551)
  line L535 (-130.7686, -181.9551) -> (-130.7954, -181.5784)
  line L536 (-130.7954, -181.5784) -> (-130.8329, -181.2168)
  line L537 (-130.8329, -181.2168) -> (-130.8812, -180.8703)
  line L538 (-130.8812, -180.8703) -> (-130.9401, -180.539)
  line L539 (-130.9401, -180.539) -> (-131.0098, -180.2228)
  line L540 (-131.0098, -180.2228) -> (-131.0902, -179.9218)
  line L541 (-131.0902, -179.9218) -> (-131.1813, -179.6359)
  line L542 (-131.1813, -179.6359) -> (-131.2832, -179.3651)
  line L543 (-131.2832, -179.3651) -> (-131.3957, -179.1095)
  line L544 (-131.3957, -179.1095) -> (-131.519, -178.869)
  line L545 (-131.519, -178.869) -> (-131.653, -178.6436)
  line L546 (-131.653, -178.6436) -> (-131.7977, -178.4334)
  line L547 (-131.7977, -178.4334) -> (-131.9524, -178.238)
  line L548 (-131.9524, -178.238) -> (-132.1163, -178.0569)
  line L549 (-132.1163, -178.0569) -> (-132.2892, -177.8901)
  line L550 (-132.2892, -177.8901) -> (-132.4712, -177.7376)
  line L551 (-132.4712, -177.7376) -> (-132.6622, -177.5995)
  line L552 (-132.6622, -177.5995) -> (-132.8624, -177.4756)
  line L553 (-132.8624, -177.4756) -> (-133.0716, -177.3661)
  line L554 (-133.0716, -177.3661) -> (-133.29, -177.2709)
  line L555 (-133.29, -177.2709) -> (-133.5174, -177.1901)
  line L556 (-133.5174, -177.1901) -> (-133.7538, -177.1235)
  line L557 (-150.1777, -175.0425) -> (-150.1777, -177.3465)
  line L558 (-150.1777, -188.403) -> (-150.1777, -190.6412)
  line L559 (-135.7538, -188.417) -> (-135.7538, -190.63)
  line L560 (-135.7538, -174.8805) -> (-135.7538, -177.0885)
  line L561 (-148.1777, -190.5636) -> (-148.1777, -188.0946)
  line L562 (-148.1777, -177.3478) -> (-148.1777, -174.8404)
  line L563 (-133.7538, -177.1235) -> (-133.7538, -174.8985)
  line L564 (-133.7538, -190.6098) -> (-133.7538, -188.3813)
  line L565 (-39.5, -192.25) -> (-193, -192.25) construction
  line L566 (-193, -192.25) -> (-193, -177.25) construction
  dimension "d105" = 47
  dimension "d106" = 15
  constraints: 1132 end point, 2 perpendicular, 1 tangent
  measures "d105" distance from line of L0 L565.end
  measures "d106" distance of L565.end L566.end
extrude "Extrusión11" cut sketch "Boceto16" against normal through all
body "Solid1"
